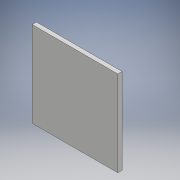
# Autodesk Inventor part: podstawa
Saved by Autodesk Inventor 2017 (Build 210142000, 142)
## iProperties
Created: 2017-05-09
Part Number: podstawa
Material: Ogólny
Document SubType Name: Modeling
Designer: Damian
Density: 1 g/cm^3
Appearance: Domyślna
Author: Damian
Autodesk Inventor part; units mm, degrees
ref_plane "YZ Plane" through (0, 0, 0) normal (1, 0, 0) x (0, 1, 0)
ref_plane "XZ Plane" through (0, 0, 0) normal (0, 1, 0) x (-1, 0, 0)
ref_plane "XY Plane" through (0, 0, 0) normal (0, 0, 1) x (1, 0, 0)
sketch "Szkic1" plane through (0, 0, 0) normal (0, 1, 0) x (-1, 0, 0)
  line L0 (-50, 50) -> (50, 50)
  line L1 (50, 50) -> (50, -50)
  line L2 (50, -50) -> (-50, -50)
  line L3 (-50, -50) -> (-50, 50)
  line L4 (-50, 50) -> (50, -50) construction
  line L5 (50, 50) -> (-50, -50) construction
  point P0 (0, 0)
  dimension "d0" = 100
  dimension "d1" = 100
  constraints: 12 end point, 2 midpoint, 2 parallel, 1 horizontal, 1 perpendicular
  measures "d0" distance of L1.end L2.end
  measures "d1" distance of L0.end L1.end
extrude "Wyciągnięcie proste1" add sketch "Szkic1" along normal blind 5
sketch "Szkic2" plane through (0, 5, 0) normal (0, 1, 0) x (1, 0, 0)
  line L0 (10, 0) -> (-10, 0)
  line L1 (-10, 0) -> (-10, -5)
  line L2 (-10, -5) -> (10, -5)
  line L3 (10, -5) -> (10, 0)
  point P0 (0, 0)
  dimension "d4" = 20
  dimension "d5" = 10
  dimension "d6" = 5
  dimension "d7" = 0
  constraints: 8 end point, 2 parallel, 1 horizontal, 1 perpendicular
  measures "d4" distance of L1.end L2.end
  measures "d5" distance from line of point (0, 0) L3
  measures "d6" distance of L2.end L0.start
  measures "d7" distance from line of point (0, 0) L0
extrude "Wyciągnięcie proste2" add sketch "Szkic2" along normal blind 30
fillet "Zaokrąglenie1" radius 10 1 edges at (10, 35, 2.5)
fillet "Zaokrąglenie2" radius 10 1 edges at (-10, 35, 2.5)
sketch "Szkic3" plane through (-10, 5, 5) normal (0, 0, 1) x (1, 0, 0)
  arc A0 (20, 20) -> (0, 20) centre (10, 20) ccw projected
  point P0 (10, -5)
  constraints: 1 coincident
hole "Otwór1" at (0, 25, 5) direction (0, 0, -1) diameter 3.2 end through all
